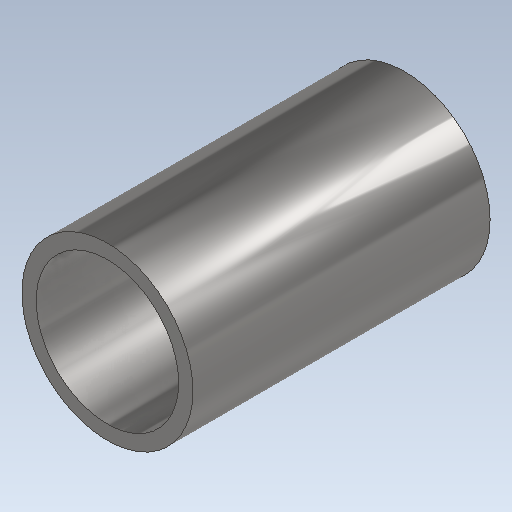
# Autodesk Inventor part: BBSleeve73.42
Saved by Autodesk Inventor 2021 (Build 250183000, 183)
## iProperties
RuleStatus: InUse
Created: 2020-04-29
Part Number: BBSleeve73.42
Material: Steel, Mild
Document SubType Name: Modeling
Designer: Hannah
Density: 7.85 g/cm^3
Appearance: Semi-Polished
Mass: 242.589 g
Surface Area: 185.056 cm^2
Volume: 30.9031 cm^3
Description: bottom bracket
Catalog Web Link: https://www.framebuilding.com/NEWPARTSPAGES/Other%20BB%20shells.htm
Vendor: Ceeway
OD: 42.0
Length: 73.0
Size: [7]
Author: Hannah
Revision Number: 1
Autodesk Inventor part; units mm, degrees
ref_plane "YZ Plane" through (0, 0, 0) normal (1, 0, 0) x (0, 1, 0)
ref_plane "XZ Plane" through (0, 0, 0) normal (0, 1, 0) x (-1, 0, 0)
ref_plane "XY Plane" through (0, 0, 0) normal (0, 0, 1) x (1, 0, 0)
sketch "Sketch1" plane through (0, 0, 0) normal (0, 0, 1) x (1, 0, 0)
  circle A0 centre (0, 0) radius 17.5
  circle A1 centre (0, 0) radius 21
  dimension "d0" = 35
  dimension "OD" = 42
  constraints: 2 centre point, 2 coincident
  measures "d0" diameter of A0
  measures "OD" diameter of A1
extrude "Extrusion1" add sketch "Sketch1" along normal mid plane 73
body "Solid1"
